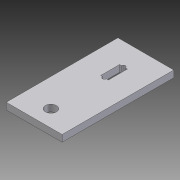
# Autodesk Inventor part: TOP
Saved by Autodesk Inventor 2012 SP2 (Build 160219200, 219)
## iProperties
Created: 2013-03-12
Part Number: TOP
Material: Default
Document SubType Name: Modeling
Designer: blacki
Density: 1 g/cm^3
Author: blacki
Autodesk Inventor part; units mm, degrees
ref_plane "YZ Plane" through (0, 0, 0) normal (1, 0, 0) x (0, 1, 0)
ref_plane "XZ Plane" through (0, 0, 0) normal (0, 1, 0) x (-1, 0, 0)
ref_plane "XY Plane" through (0, 0, 0) normal (0, 0, 1) x (1, 0, 0)
sketch "Sketch1" plane through (0, 0, 0) normal (0, 0, 1) x (1, 0, 0)
  line L0 (-25, 50) -> (25, 50)
  line L1 (25, 50) -> (25, -50)
  line L2 (25, -50) -> (-25, -50)
  line L3 (-25, -50) -> (-25, 50)
  line L4 (-25, 0) -> (25, 0) construction
  point P0 (0, 0)
  point P1 (0, 0)
  dimension "d0" = 50
  dimension "d1" = 100
  constraints: 10 end point, 3 midpoint, 2 parallel, 1 coincident, 1 horizontal, 1 perpendicular
  measures "d0" distance of L1.end L2.end
  measures "d1" distance of L0.end L1.end
extrude "Extrusion1" add sketch "Sketch1" along normal blind 6
sketch "Sketch2" plane through (0, 0, 6) normal (0, 0, 1) x (1, 0, 0)
  line L0 (-25, 50) -> (25, 50) projected
  line L1 (25, -50) -> (-25, -50) projected
  line L2 (0, 50) -> (0, -35) construction
  point P0 (0, 0)
  dimension "d4" = 15
  constraints: 2 end point, 1 coincident, 1 midpoint, 1 perpendicular
  measures "d4" distance from line of L1 L2.end
hole "Hole1" at (0, -35, 6) direction (0, 0, -1) diameter 10 end through all
sketch "Sketch3" plane through (0, 0, 6) normal (0, 0, 1) x (1, 0, 0)
  line L0 (-25, 50) -> (25, 50) projected
  line L1 (-3.5, 30) -> (3.5, 30)
  line L2 (3.5, 30) -> (3.5, 13)
  line L3 (3.5, 13) -> (-3.5, 13)
  line L4 (-3.5, 13) -> (-3.5, 30)
  line L5 (0, 30) -> (0, 13) construction
  circle A0 centre (0, 30) radius 1.75
  circle A1 centre (0, 13) radius 1.75
  point P0 (0, 0)
  dimension "d12" = 7
  dimension "d13" = 17
  dimension "d14" = 3.5
  dimension "d15" = 3.5
  dimension "d16" = 20
  constraints: 10 end point, 2 centre point, 2 coincident, 2 midpoint, 2 parallel, 1 horizontal, 1 perpendicular, 1 point on line
  measures "d12" distance of L2.end L3.end
  measures "d13" distance of L1.end L2.end
  measures "d14" diameter of A0
  measures "d15" diameter of A1
  measures "d16" distance between parallel lines of L0 L1
extrude "Extrusion2" cut sketch "Sketch3" against normal up to next
sketch "Sketch4" plane through (0, 0, 6) normal (0, 0, 1) x (1, 0, 0)
  arc A0 (1.75, 30) -> (-1.75, 30) centre (0, 30) ccw projected
  line L0 (-25, 50) -> (25, 50) projected
  line L1 (-25, -50) -> (-25, 50) projected
  line L2 (10, 44) -> (25, 44) projected
  line L3 (25, 50) -> (25, 44) projected
  line L4 (10, 50) -> (25, 50) projected
  line L5 (10, 50) -> (10, 44) projected
  line L6 (-25, 44) -> (-10, 44) projected
  line L7 (-10, 50) -> (-10, 44) projected
  line L8 (-25, 50) -> (-10, 50) projected
  line L9 (-25, 50) -> (-25, 44) projected
  line L10 (0, 50) -> (0, 31.75) construction
  point P0 (0, 0)
  constraints: 2 end point, 1 midpoint, 1 point on circle
extrude "Extrusion3" cut sketch "Sketch4" against normal up to next
body "Solid1"
